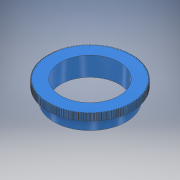
# Autodesk Inventor part: タミヤダンパー部品4
Saved by Autodesk Inventor 2020.1 (Build 241239000, 239)
## iProperties
Created: 2018-09-17
Part Number: タミヤダンパー部品4
Material: 一般
Document SubType Name: Modeling
Designer: 杉本　賢二郎
Density: 1 g/cm^3
Appearance: 既定
Author: 杉本　賢二郎
Autodesk Inventor part; units mm, degrees
(part 1 of 2)
ref_plane "YZ Plane" through (0, 0, 0) normal (1, 0, 0) x (0, 1, 0)
ref_plane "XZ Plane" through (0, 0, 0) normal (0, 1, 0) x (-1, 0, 0)
ref_plane "XY Plane" through (0, 0, 0) normal (0, 0, 1) x (1, 0, 0)
sketch "スケッチ1" plane through (0, 0, 0) normal (0, 1, 0) x (-1, 0, 0)
  line L0 (6.6972, 6.0123) -> (6.6034, 5.8356)
  arc A0 (6.8569, 5.8295) -> (6.6972, 6.0123) centre (0, 0) ccw
  line L1 (6.6692, 5.7603) -> (6.8569, 5.8295)
  arc A1 (6.6692, 5.7603) -> (6.6034, 5.8356) centre (0, 0) ccw
  line L2 (6.4207, 6.3067) -> (6.335, 6.126)
  arc A2 (6.5885, 6.1313) -> (6.4207, 6.3067) centre (0, 0) ccw
  line L3 (6.4041, 6.0538) -> (6.5885, 6.1313)
  arc A3 (6.4041, 6.0538) -> (6.335, 6.126) centre (0, 0) ccw
  line L4 (6.1313, 6.5885) -> (6.0538, 6.4041)
  arc A4 (6.3067, 6.4207) -> (6.1313, 6.5885) centre (0, 0) ccw
  line L5 (6.126, 6.335) -> (6.3067, 6.4207)
  arc A5 (6.126, 6.335) -> (6.0538, 6.4041) centre (0, 0) ccw
  line L6 (5.8295, 6.8569) -> (5.7603, 6.6692)
  arc A6 (6.0123, 6.6972) -> (5.8295, 6.8569) centre (0, 0) ccw
  line L7 (5.8356, 6.6034) -> (6.0123, 6.6972)
  arc A7 (5.8356, 6.6034) -> (5.7603, 6.6692) centre (0, 0) ccw
  line L8 (5.516, 7.1115) -> (5.4553, 6.921)
  arc A8 (5.7058, 6.9602) -> (5.516, 7.1115) centre (0, 0) ccw
  line L9 (5.5335, 6.8586) -> (5.7058, 6.9602)
  arc A9 (5.5335, 6.8586) -> (5.4553, 6.921) centre (0, 0) ccw
  line L10 (5.1914, 7.3518) -> (5.1393, 7.1587)
  arc A10 (5.3878, 7.2091) -> (5.1914, 7.3518) centre (0, 0) ccw
  line L11 (5.2202, 7.1) -> (5.3878, 7.2091)
  arc A11 (5.2202, 7.1) -> (5.1393, 7.1587) centre (0, 0) ccw
  line L12 (4.8563, 7.5774) -> (4.813, 7.3821)
  arc A12 (5.0589, 7.4436) -> (4.8563, 7.5774) centre (0, 0) ccw
  line L13 (4.8964, 7.327) -> (5.0589, 7.4436)
  arc A13 (4.8964, 7.327) -> (4.813, 7.3821) centre (0, 0) ccw
  line L14 (4.5115, 7.7876) -> (4.4769, 7.5906)
  arc A14 (4.7199, 7.6631) -> (4.5115, 7.7876) centre (0, 0) ccw
  line L15 (4.5628, 7.5393) -> (4.7199, 7.6631)
  arc A15 (4.5628, 7.5393) -> (4.4769, 7.5906) centre (0, 0) ccw
  line L16 (4.1575, 7.9822) -> (4.1319, 7.7838)
  arc A16 (4.3713, 7.8671) -> (4.1575, 7.9822) centre (0, 0) ccw
  line L17 (4.2199, 7.7364) -> (4.3713, 7.8671)
  arc A17 (4.2199, 7.7364) -> (4.1319, 7.7838) centre (0, 0) ccw
  line L18 (3.7952, 8.1607) -> (3.7785, 7.9614)
  arc A18 (4.014, 8.0553) -> (3.7952, 8.1607) centre (0, 0) ccw
  line L19 (3.8686, 7.918) -> (4.014, 8.0553)
  arc A19 (3.8686, 7.918) -> (3.7785, 7.9614) centre (0, 0) ccw
  line L20 (3.4253, 8.3227) -> (3.4175, 8.1229)
  arc A20 (3.6485, 8.2273) -> (3.4253, 8.3227) centre (0, 0) ccw
  line L21 (3.5095, 8.0836) -> (3.6485, 8.2273)
  arc A21 (3.5095, 8.0836) -> (3.4175, 8.1229) centre (0, 0) ccw
  line L22 (3.0484, 8.468) -> (3.0496, 8.268)
  arc A22 (3.2757, 8.3827) -> (3.0484, 8.468) centre (0, 0) ccw
  line L23 (3.1433, 8.2329) -> (3.2757, 8.3827)
  arc A23 (3.1433, 8.2329) -> (3.0496, 8.268) centre (0, 0) ccw
  line L24 (2.6654, 8.5962) -> (2.6756, 8.3965)
  arc A24 (2.8964, 8.5212) -> (2.6654, 8.5962) centre (0, 0) ccw
  line L25 (2.7707, 8.3656) -> (2.8964, 8.5212)
  arc A25 (2.7707, 8.3656) -> (2.6756, 8.3965) centre (0, 0) ccw
  line L26 (2.2771, 8.7072) -> (2.2962, 8.5081)
  arc A26 (2.5111, 8.6426) -> (2.2771, 8.7072) centre (0, 0) ccw
  line L27 (2.3926, 8.4815) -> (2.5111, 8.6426)
  arc A27 (2.3926, 8.4815) -> (2.2962, 8.5081) centre (0, 0) ccw
  line L28 (1.8842, 8.8006) -> (1.9122, 8.6025)
  arc A28 (2.1209, 8.7465) -> (1.8842, 8.8006) centre (0, 0) ccw
  line L29 (2.0097, 8.5803) -> (2.1209, 8.7465)
  arc A29 (2.0097, 8.5803) -> (1.9122, 8.6025) centre (0, 0) ccw
  line L30 (1.4874, 8.8762) -> (1.5243, 8.6797)
  arc A30 (1.7263, 8.8329) -> (1.4874, 8.8762) centre (0, 0) ccw
  line L31 (1.6227, 8.6618) -> (1.7263, 8.8329)
  arc A31 (1.6227, 8.6618) -> (1.5243, 8.6797) centre (0, 0) ccw
  line L32 (1.0877, 8.934) -> (1.1334, 8.7393)
  arc A32 (1.3283, 8.9014) -> (1.0877, 8.934) centre (0, 0) ccw
  line L33 (1.2325, 8.7259) -> (1.3283, 8.9014)
  arc A33 (1.2325, 8.7259) -> (1.1334, 8.7393) centre (0, 0) ccw
  line L34 (0.6858, 8.9738) -> (0.7401, 8.7814)
  arc A34 (0.9276, 8.9521) -> (0.6858, 8.9738) centre (0, 0) ccw
  line L35 (0.8397, 8.7724) -> (0.9276, 8.9521)
  arc A35 (0.8397, 8.7724) -> (0.7401, 8.7814) centre (0, 0) ccw
  line L36 (0.2825, 8.9956) -> (0.3454, 8.8057)
  arc A36 (0.525, 8.9847) -> (0.2825, 8.9956) centre (0, 0) ccw
  line L37 (0.4453, 8.8012) -> (0.525, 8.9847)
  arc A37 (0.4453, 8.8012) -> (0.3454, 8.8057) centre (0, 0) ccw
  line L38 (-0.1214, 8.9992) -> (-0.05, 8.8124)
  arc A38 (0.1214, 8.9992) -> (-0.1214, 8.9992) centre (0, 0) ccw
  line L39 (0.05, 8.8124) -> (0.1214, 8.9992)
  arc A39 (0.05, 8.8124) -> (-0.05, 8.8124) centre (0, 0) ccw
  line L40 (-0.525, 8.9847) -> (-0.4453, 8.8012)
  arc A40 (-0.2825, 8.9956) -> (-0.525, 8.9847) centre (0, 0) ccw
  line L41 (-0.3454, 8.8057) -> (-0.2825, 8.9956)
  arc A41 (-0.3454, 8.8057) -> (-0.4453, 8.8012) centre (0, 0) ccw
  line L42 (-0.9276, 8.9521) -> (-0.8397, 8.7724)
  arc A42 (-0.6858, 8.9738) -> (-0.9276, 8.9521) centre (0, 0) ccw
  line L43 (-0.7401, 8.7814) -> (-0.6858, 8.9738)
  arc A43 (-0.7401, 8.7814) -> (-0.8397, 8.7724) centre (0, 0) ccw
  line L44 (-1.3283, 8.9014) -> (-1.2325, 8.7259)
  arc A44 (-1.0877, 8.934) -> (-1.3283, 8.9014) centre (0, 0) ccw
  line L45 (-1.1334, 8.7393) -> (-1.0877, 8.934)
  arc A45 (-1.1334, 8.7393) -> (-1.2325, 8.7259) centre (0, 0) ccw
  line L46 (-1.7263, 8.8329) -> (-1.6227, 8.6618)
  arc A46 (-1.4874, 8.8762) -> (-1.7263, 8.8329) centre (0, 0) ccw
  line L47 (-1.5243, 8.6797) -> (-1.4874, 8.8762)
  arc A47 (-1.5243, 8.6797) -> (-1.6227, 8.6618) centre (0, 0) ccw
  line L48 (-2.1209, 8.7465) -> (-2.0097, 8.5803)
  arc A48 (-1.8842, 8.8006) -> (-2.1209, 8.7465) centre (0, 0) ccw
  line L49 (-1.9122, 8.6025) -> (-1.8842, 8.8006)
  arc A49 (-1.9122, 8.6025) -> (-2.0097, 8.5803) centre (0, 0) ccw
  line L50 (-2.5111, 8.6426) -> (-2.3926, 8.4815)
  arc A50 (-2.2771, 8.7072) -> (-2.5111, 8.6426) centre (0, 0) ccw
  line L51 (-2.2962, 8.5081) -> (-2.2771, 8.7072)
  arc A51 (-2.2962, 8.5081) -> (-2.3926, 8.4815) centre (0, 0) ccw
  line L52 (-2.8964, 8.5212) -> (-2.7707, 8.3656)
  arc A52 (-2.6654, 8.5962) -> (-2.8964, 8.5212) centre (0, 0) ccw
  line L53 (-2.6756, 8.3965) -> (-2.6654, 8.5962)
  arc A53 (-2.6756, 8.3965) -> (-2.7707, 8.3656) centre (0, 0) ccw
  line L54 (-3.2757, 8.3827) -> (-3.1433, 8.2329)
  arc A54 (-3.0484, 8.468) -> (-3.2757, 8.3827) centre (0, 0) ccw
  line L55 (-3.0496, 8.268) -> (-3.0484, 8.468)
  arc A55 (-3.0496, 8.268) -> (-3.1433, 8.2329) centre (0, 0) ccw
  line L56 (-3.6485, 8.2273) -> (-3.5095, 8.0836)
  arc A56 (-3.4253, 8.3227) -> (-3.6485, 8.2273) centre (0, 0) ccw
  line L57 (-3.4175, 8.1229) -> (-3.4253, 8.3227)
  arc A57 (-3.4175, 8.1229) -> (-3.5095, 8.0836) centre (0, 0) ccw
  line L58 (-4.014, 8.0553) -> (-3.8686, 7.918)
  arc A58 (-3.7952, 8.1607) -> (-4.014, 8.0553) centre (0, 0) ccw
  line L59 (-3.7785, 7.9614) -> (-3.7952, 8.1607)
  arc A59 (-3.7785, 7.9614) -> (-3.8686, 7.918) centre (0, 0) ccw
  line L60 (-4.3713, 7.8671) -> (-4.2199, 7.7364)
  arc A60 (-4.1575, 7.9822) -> (-4.3713, 7.8671) centre (0, 0) ccw
  line L61 (-4.1319, 7.7838) -> (-4.1575, 7.9822)
  arc A61 (-4.1319, 7.7838) -> (-4.2199, 7.7364) centre (0, 0) ccw
  line L62 (-4.7199, 7.6631) -> (-4.5628, 7.5393)
  arc A62 (-4.5115, 7.7876) -> (-4.7199, 7.6631) centre (0, 0) ccw
  line L63 (-4.4769, 7.5906) -> (-4.5115, 7.7876)
  arc A63 (-4.4769, 7.5906) -> (-4.5628, 7.5393) centre (0, 0) ccw
  line L64 (-5.0589, 7.4436) -> (-4.8964, 7.327)
  arc A64 (-4.8563, 7.5774) -> (-5.0589, 7.4436) centre (0, 0) ccw
  line L65 (-4.813, 7.3821) -> (-4.8563, 7.5774)
  arc A65 (-4.813, 7.3821) -> (-4.8964, 7.327) centre (0, 0) ccw
  line L66 (-5.3878, 7.2091) -> (-5.2202, 7.1)
  arc A66 (-5.1914, 7.3518) -> (-5.3878, 7.2091) centre (0, 0) ccw
  line L67 (-5.1393, 7.1587) -> (-5.1914, 7.3518)
  arc A67 (-5.1393, 7.1587) -> (-5.2202, 7.1) centre (0, 0) ccw
  line L68 (-5.7058, 6.9602) -> (-5.5335, 6.8586)
  arc A68 (-5.516, 7.1115) -> (-5.7058, 6.9602) centre (0, 0) ccw
  line L69 (-5.4553, 6.921) -> (-5.516, 7.1115)
  arc A69 (-5.4553, 6.921) -> (-5.5335, 6.8586) centre (0, 0) ccw
  line L70 (-6.0123, 6.6972) -> (-5.8356, 6.6034)
  arc A70 (-5.8295, 6.8569) -> (-6.0123, 6.6972) centre (0, 0) ccw
  line L71 (-5.7603, 6.6692) -> (-5.8295, 6.8569)
  arc A71 (-5.7603, 6.6692) -> (-5.8356, 6.6034) centre (0, 0) ccw
  line L72 (-6.3067, 6.4207) -> (-6.126, 6.335)
  arc A72 (-6.1313, 6.5885) -> (-6.3067, 6.4207) centre (0, 0) ccw
  line L73 (-6.0538, 6.4041) -> (-6.1313, 6.5885)
  arc A73 (-6.0538, 6.4041) -> (-6.126, 6.335) centre (0, 0) ccw
  line L74 (-6.5885, 6.1313) -> (-6.4041, 6.0538)
  arc A74 (-6.4207, 6.3067) -> (-6.5885, 6.1313) centre (0, 0) ccw
  line L75 (-6.335, 6.126) -> (-6.4207, 6.3067)
  arc A75 (-6.335, 6.126) -> (-6.4041, 6.0538) centre (0, 0) ccw
  line L76 (-6.8569, 5.8295) -> (-6.6692, 5.7603)
  arc A76 (-6.6972, 6.0123) -> (-6.8569, 5.8295) centre (0, 0) ccw
  line L77 (-6.6034, 5.8356) -> (-6.6972, 6.0123)
  arc A77 (-6.6034, 5.8356) -> (-6.6692, 5.7603) centre (0, 0) ccw
  line L78 (7.5774, -4.8563) -> (7.3821, -4.813)
  arc A78 (7.4436, -5.0589) -> (7.5774, -4.8563) centre (0, 0) ccw
  line L79 (7.327, -4.8964) -> (7.4436, -5.0589)
  arc A79 (7.327, -4.8964) -> (7.3821, -4.813) centre (0, 0) ccw
  line L80 (7.7876, -4.5115) -> (7.5906, -4.4769)
  arc A80 (7.6631, -4.7199) -> (7.7876, -4.5115) centre (0, 0) ccw
  line L81 (7.5393, -4.5628) -> (7.6631, -4.7199)
  arc A81 (7.5393, -4.5628) -> (7.5906, -4.4769) centre (0, 0) ccw
  line L82 (7.9822, -4.1575) -> (7.7838, -4.1319)
  arc A82 (7.8671, -4.3713) -> (7.9822, -4.1575) centre (0, 0) ccw
  line L83 (7.7364, -4.2199) -> (7.8671, -4.3713)
  arc A83 (7.7364, -4.2199) -> (7.7838, -4.1319) centre (0, 0) ccw
  line L84 (8.1607, -3.7952) -> (7.9614, -3.7785)
  arc A84 (8.0553, -4.014) -> (8.1607, -3.7952) centre (0, 0) ccw
  line L85 (7.918, -3.8686) -> (8.0553, -4.014)
  arc A85 (7.918, -3.8686) -> (7.9614, -3.7785) centre (0, 0) ccw
  line L86 (8.3227, -3.4253) -> (8.1229, -3.4175)
  arc A86 (8.2273, -3.6485) -> (8.3227, -3.4253) centre (0, 0) ccw
  line L87 (8.0836, -3.5095) -> (8.2273, -3.6485)
  arc A87 (8.0836, -3.5095) -> (8.1229, -3.4175) centre (0, 0) ccw
  line L88 (8.468, -3.0484) -> (8.268, -3.0496)
  arc A88 (8.3827, -3.2757) -> (8.468, -3.0484) centre (0, 0) ccw
  line L89 (8.2329, -3.1433) -> (8.3827, -3.2757)
  arc A89 (8.2329, -3.1433) -> (8.268, -3.0496) centre (0, 0) ccw
  line L90 (8.5962, -2.6654) -> (8.3965, -2.6756)
  arc A90 (8.5212, -2.8964) -> (8.5962, -2.6654) centre (0, 0) ccw
  line L91 (8.3656, -2.7707) -> (8.5212, -2.8964)
  arc A91 (8.3656, -2.7707) -> (8.3965, -2.6756) centre (0, 0) ccw
  line L92 (8.7072, -2.2771) -> (8.5081, -2.2962)
  arc A92 (8.6426, -2.5111) -> (8.7072, -2.2771) centre (0, 0) ccw
  line L93 (8.4815, -2.3926) -> (8.6426, -2.5111)
  arc A93 (8.4815, -2.3926) -> (8.5081, -2.2962) centre (0, 0) ccw
  line L94 (8.8006, -1.8842) -> (8.6025, -1.9122)
  arc A94 (8.7465, -2.1209) -> (8.8006, -1.8842) centre (0, 0) ccw
  line L95 (8.5803, -2.0097) -> (8.7465, -2.1209)
  arc A95 (8.5803, -2.0097) -> (8.6025, -1.9122) centre (0, 0) ccw
  line L96 (8.8762, -1.4874) -> (8.6797, -1.5243)
  arc A96 (8.8329, -1.7263) -> (8.8762, -1.4874) centre (0, 0) ccw
  line L97 (8.6618, -1.6227) -> (8.8329, -1.7263)
  arc A97 (8.6618, -1.6227) -> (8.6797, -1.5243) centre (0, 0) ccw
  line L98 (8.934, -1.0877) -> (8.7393, -1.1334)
  arc A98 (8.9014, -1.3283) -> (8.934, -1.0877) centre (0, 0) ccw
  line L99 (8.7259, -1.2325) -> (8.9014, -1.3283)
  arc A99 (8.7259, -1.2325) -> (8.7393, -1.1334) centre (0, 0) ccw
  line L100 (8.9738, -0.6858) -> (8.7814, -0.7401)
  arc A100 (8.9521, -0.9276) -> (8.9738, -0.6858) centre (0, 0) ccw
  line L101 (8.7724, -0.8397) -> (8.9521, -0.9276)
  arc A101 (8.7724, -0.8397) -> (8.7814, -0.7401) centre (0, 0) ccw
  line L102 (8.9956, -0.2825) -> (8.8057, -0.3454)
  arc A102 (8.9847, -0.525) -> (8.9956, -0.2825) centre (0, 0) ccw
  line L103 (8.8012, -0.4453) -> (8.9847, -0.525)
  arc A103 (8.8012, -0.4453) -> (8.8057, -0.3454) centre (0, 0) ccw
  line L104 (8.9992, 0.1214) -> (8.8124, 0.05)
  arc A104 (8.9992, -0.1214) -> (8.9992, 0.1214) centre (0, 0) ccw
  line L105 (8.8124, -0.05) -> (8.9992, -0.1214)
  arc A105 (8.8124, -0.05) -> (8.8124, 0.05) centre (0, 0) ccw
  line L106 (8.9847, 0.525) -> (8.8012, 0.4453)
  arc A106 (8.9956, 0.2825) -> (8.9847, 0.525) centre (0, 0) ccw
  line L107 (8.8057, 0.3454) -> (8.9956, 0.2825)
  arc A107 (8.8057, 0.3454) -> (8.8012, 0.4453) centre (0, 0) ccw
  line L108 (8.9521, 0.9276) -> (8.7724, 0.8397)
  arc A108 (8.9738, 0.6858) -> (8.9521, 0.9276) centre (0, 0) ccw
  line L109 (8.7814, 0.7401) -> (8.9738, 0.6858)
  arc A109 (8.7814, 0.7401) -> (8.7724, 0.8397) centre (0, 0) ccw
  line L110 (8.9014, 1.3283) -> (8.7259, 1.2325)
  arc A110 (8.934, 1.0877) -> (8.9014, 1.3283) centre (0, 0) ccw
  line L111 (8.7393, 1.1334) -> (8.934, 1.0877)
  arc A111 (8.7393, 1.1334) -> (8.7259, 1.2325) centre (0, 0) ccw
  line L112 (8.8329, 1.7263) -> (8.6618, 1.6227)
  arc A112 (8.8762, 1.4874) -> (8.8329, 1.7263) centre (0, 0) ccw
  line L113 (8.6797, 1.5243) -> (8.8762, 1.4874)
  arc A113 (8.6797, 1.5243) -> (8.6618, 1.6227) centre (0, 0) ccw
  line L114 (8.7465, 2.1209) -> (8.5803, 2.0097)
  arc A114 (8.8006, 1.8842) -> (8.7465, 2.1209) centre (0, 0) ccw
  line L115 (8.6025, 1.9122) -> (8.8006, 1.8842)
  arc A115 (8.6025, 1.9122) -> (8.5803, 2.0097) centre (0, 0) ccw
  line L116 (8.6426, 2.5111) -> (8.4815, 2.3926)
  arc A116 (8.7072, 2.2771) -> (8.6426, 2.5111) centre (0, 0) ccw
  line L117 (8.5081, 2.2962) -> (8.7072, 2.2771)
  arc A117 (8.5081, 2.2962) -> (8.4815, 2.3926) centre (0, 0) ccw
  line L118 (8.5212, 2.8964) -> (8.3656, 2.7707)
  arc A118 (8.5962, 2.6654) -> (8.5212, 2.8964) centre (0, 0) ccw
  line L119 (8.3965, 2.6756) -> (8.5962, 2.6654)
  arc A119 (8.3965, 2.6756) -> (8.3656, 2.7707) centre (0, 0) ccw
  line L120 (8.3827, 3.2757) -> (8.2329, 3.1433)
  arc A120 (8.468, 3.0484) -> (8.3827, 3.2757) centre (0, 0) ccw
  line L121 (8.268, 3.0496) -> (8.468, 3.0484)
  arc A121 (8.268, 3.0496) -> (8.2329, 3.1433) centre (0, 0) ccw
  line L122 (8.2273, 3.6485) -> (8.0836, 3.5095)
  arc A122 (8.3227, 3.4253) -> (8.2273, 3.6485) centre (0, 0) ccw
  line L123 (8.1229, 3.4175) -> (8.3227, 3.4253)
  arc A123 (8.1229, 3.4175) -> (8.0836, 3.5095) centre (0, 0) ccw
  line L124 (8.0553, 4.014) -> (7.918, 3.8686)
  arc A124 (8.1607, 3.7952) -> (8.0553, 4.014) centre (0, 0) ccw
  line L125 (7.9614, 3.7785) -> (8.1607, 3.7952)
  arc A125 (7.9614, 3.7785) -> (7.918, 3.8686) centre (0, 0) ccw
  line L126 (7.8671, 4.3713) -> (7.7364, 4.2199)
  arc A126 (7.9822, 4.1575) -> (7.8671, 4.3713) centre (0, 0) ccw
  line L127 (7.7838, 4.1319) -> (7.9822, 4.1575)
  arc A127 (7.7838, 4.1319) -> (7.7364, 4.2199) centre (0, 0) ccw
  line L128 (7.6631, 4.7199) -> (7.5393, 4.5628)
  arc A128 (7.7876, 4.5115) -> (7.6631, 4.7199) centre (0, 0) ccw
  line L129 (7.5906, 4.4769) -> (7.7876, 4.5115)
  arc A129 (7.5906, 4.4769) -> (7.5393, 4.5628) centre (0, 0) ccw
  line L130 (7.4436, 5.0589) -> (7.327, 4.8964)
  arc A130 (7.5774, 4.8563) -> (7.4436, 5.0589) centre (0, 0) ccw
  line L131 (7.3821, 4.813) -> (7.5774, 4.8563)
  arc A131 (7.3821, 4.813) -> (7.327, 4.8964) centre (0, 0) ccw
  line L132 (7.2091, 5.3878) -> (7.1, 5.2202)
  arc A132 (7.3518, 5.1914) -> (7.2091, 5.3878) centre (0, 0) ccw
  line L133 (7.1587, 5.1393) -> (7.3518, 5.1914)
  arc A133 (7.1587, 5.1393) -> (7.1, 5.2202) centre (0, 0) ccw
  line L134 (6.9602, 5.7058) -> (6.8586, 5.5335)
  arc A134 (7.1115, 5.516) -> (6.9602, 5.7058) centre (0, 0) ccw
  line L135 (6.921, 5.4553) -> (7.1115, 5.516)
  arc A135 (6.921, 5.4553) -> (6.8586, 5.5335) centre (0, 0) ccw
  line L136 (6.6972, 6.0123) -> (6.6034, 5.8356)
  arc A136 (6.8569, 5.8295) -> (6.6972, 6.0123) centre (0, 0) ccw
  line L137 (6.6692, 5.7603) -> (6.8569, 5.8295)
  arc A137 (6.6692, 5.7603) -> (6.6034, 5.8356) centre (0, 0) ccw
  line L138 (6.4207, 6.3067) -> (6.335, 6.126)
  arc A138 (6.5885, 6.1313) -> (6.4207, 6.3067) centre (0, 0) ccw
  line L139 (6.4041, 6.0538) -> (6.5885, 6.1313)
  arc A139 (6.4041, 6.0538) -> (6.335, 6.126) centre (0, 0) ccw
  line L140 (6.1313, 6.5885) -> (6.0538, 6.4041)
  arc A140 (6.3067, 6.4207) -> (6.1313, 6.5885) centre (0, 0) ccw
  line L141 (6.126, 6.335) -> (6.3067, 6.4207)
  arc A141 (6.126, 6.335) -> (6.0538, 6.4041) centre (0, 0) ccw
  line L142 (5.8295, 6.8569) -> (5.7603, 6.6692)
  arc A142 (6.0123, 6.6972) -> (5.8295, 6.8569) centre (0, 0) ccw
  line L143 (5.8356, 6.6034) -> (6.0123, 6.6972)
  arc A143 (5.8356, 6.6034) -> (5.7603, 6.6692) centre (0, 0) ccw
  line L144 (5.516, 7.1115) -> (5.4553, 6.921)
  arc A144 (5.7058, 6.9602) -> (5.516, 7.1115) centre (0, 0) ccw
  line L145 (5.5335, 6.8586) -> (5.7058, 6.9602)
  arc A145 (5.5335, 6.8586) -> (5.4553, 6.921) centre (0, 0) ccw
  line L146 (5.1914, 7.3518) -> (5.1393, 7.1587)
  arc A146 (5.3878, 7.2091) -> (5.1914, 7.3518) centre (0, 0) ccw
  line L147 (5.2202, 7.1) -> (5.3878, 7.2091)
  arc A147 (5.2202, 7.1) -> (5.1393, 7.1587) centre (0, 0) ccw
  line L148 (4.8563, 7.5774) -> (4.813, 7.3821)
  arc A148 (5.0589, 7.4436) -> (4.8563, 7.5774) centre (0, 0) ccw
  line L149 (4.8964, 7.327) -> (5.0589, 7.4436)
  arc A149 (4.8964, 7.327) -> (4.813, 7.3821) centre (0, 0) ccw
  line L150 (4.5115, 7.7876) -> (4.4769, 7.5906)
  arc A150 (4.7199, 7.6631) -> (4.5115, 7.7876) centre (0, 0) ccw
  line L151 (4.5628, 7.5393) -> (4.7199, 7.6631)
  arc A151 (4.5628, 7.5393) -> (4.4769, 7.5906) centre (0, 0) ccw
  line L152 (4.1575, 7.9822) -> (4.1319, 7.7838)
  arc A152 (4.3713, 7.8671) -> (4.1575, 7.9822) centre (0, 0) ccw
  line L153 (4.2199, 7.7364) -> (4.3713, 7.8671)
  arc A153 (4.2199, 7.7364) -> (4.1319, 7.7838) centre (0, 0) ccw
  line L154 (3.7952, 8.1607) -> (3.7785, 7.9614)
  line L155 (3.8686, 7.918) -> (4.014, 8.0553)
  arc A154 (3.8686, 7.918) -> (3.7785, 7.9614) centre (0, 0) ccw
  line L156 (1.7263, -8.8329) -> (1.6227, -8.6618)
  arc A155 (1.4874, -8.8762) -> (1.7263, -8.8329) centre (0, 0) ccw
  line L157 (1.5243, -8.6797) -> (1.4874, -8.8762)
  arc A156 (1.5243, -8.6797) -> (1.6227, -8.6618) centre (0, 0) ccw
  line L158 (2.1209, -8.7465) -> (2.0097, -8.5803)
  arc A157 (1.8842, -8.8006) -> (2.1209, -8.7465) centre (0, 0) ccw
  line L159 (1.9122, -8.6025) -> (1.8842, -8.8006)
  arc A158 (1.9122, -8.6025) -> (2.0097, -8.5803) centre (0, 0) ccw
  line L160 (2.5111, -8.6426) -> (2.3926, -8.4815)
  arc A159 (2.2771, -8.7072) -> (2.5111, -8.6426) centre (0, 0) ccw
  line L161 (2.2962, -8.5081) -> (2.2771, -8.7072)
  arc A160 (2.2962, -8.5081) -> (2.3926, -8.4815) centre (0, 0) ccw
  line L162 (2.8964, -8.5212) -> (2.7707, -8.3656)
  arc A161 (2.6654, -8.5962) -> (2.8964, -8.5212) centre (0, 0) ccw
  line L163 (2.6756, -8.3965) -> (2.6654, -8.5962)
  arc A162 (2.6756, -8.3965) -> (2.7707, -8.3656) centre (0, 0) ccw
  line L164 (3.2757, -8.3827) -> (3.1433, -8.2329)
  arc A163 (3.0484, -8.468) -> (3.2757, -8.3827) centre (0, 0) ccw
  line L165 (3.0496, -8.268) -> (3.0484, -8.468)
  arc A164 (3.0496, -8.268) -> (3.1433, -8.2329) centre (0, 0) ccw
  line L166 (3.6485, -8.2273) -> (3.5095, -8.0836)
  arc A165 (3.4253, -8.3227) -> (3.6485, -8.2273) centre (0, 0) ccw
  line L167 (3.4175, -8.1229) -> (3.4253, -8.3227)
  arc A166 (3.4175, -8.1229) -> (3.5095, -8.0836) centre (0, 0) ccw
  line L168 (4.014, -8.0553) -> (3.8686, -7.918)
  arc A167 (3.7952, -8.1607) -> (4.014, -8.0553) centre (0, 0) ccw
  line L169 (3.7785, -7.9614) -> (3.7952, -8.1607)
  arc A168 (3.7785, -7.9614) -> (3.8686, -7.918) centre (0, 0) ccw
  line L170 (4.3713, -7.8671) -> (4.2199, -7.7364)
  arc A169 (4.1575, -7.9822) -> (4.3713, -7.8671) centre (0, 0) ccw
  line L171 (4.1319, -7.7838) -> (4.1575, -7.9822)
  arc A170 (4.1319, -7.7838) -> (4.2199, -7.7364) centre (0, 0) ccw
  line L172 (4.7199, -7.6631) -> (4.5628, -7.5393)
  arc A171 (4.5115, -7.7876) -> (4.7199, -7.6631) centre (0, 0) ccw
  line L173 (4.4769, -7.5906) -> (4.5115, -7.7876)
  arc A172 (4.4769, -7.5906) -> (4.5628, -7.5393) centre (0, 0) ccw
  line L174 (5.0589, -7.4436) -> (4.8964, -7.327)
  arc A173 (4.8563, -7.5774) -> (5.0589, -7.4436) centre (0, 0) ccw
  line L175 (4.813, -7.3821) -> (4.8563, -7.5774)
  arc A174 (4.813, -7.3821) -> (4.8964, -7.327) centre (0, 0) ccw
  line L176 (5.3878, -7.2091) -> (5.2202, -7.1)
  arc A175 (5.1914, -7.3518) -> (5.3878, -7.2091) centre (0, 0) ccw
  line L177 (5.1393, -7.1587) -> (5.1914, -7.3518)
  arc A176 (5.1393, -7.1587) -> (5.2202, -7.1) centre (0, 0) ccw
  line L178 (5.7058, -6.9602) -> (5.5335, -6.8586)
  arc A177 (5.516, -7.1115) -> (5.7058, -6.9602) centre (0, 0) ccw
  line L179 (5.4553, -6.921) -> (5.516, -7.1115)
  arc A178 (5.4553, -6.921) -> (5.5335, -6.8586) centre (0, 0) ccw
  line L180 (6.0123, -6.6972) -> (5.8356, -6.6034)
  arc A179 (5.8295, -6.8569) -> (6.0123, -6.6972) centre (0, 0) ccw
  line L181 (5.7603, -6.6692) -> (5.8295, -6.8569)
  arc A180 (5.7603, -6.6692) -> (5.8356, -6.6034) centre (0, 0) ccw
  line L182 (6.3067, -6.4207) -> (6.126, -6.335)
  arc A181 (6.1313, -6.5885) -> (6.3067, -6.4207) centre (0, 0) ccw
  line L183 (6.0538, -6.4041) -> (6.1313, -6.5885)
  arc A182 (6.0538, -6.4041) -> (6.126, -6.335) centre (0, 0) ccw
  line L184 (6.5885, -6.1313) -> (6.4041, -6.0538)
  arc A183 (6.4207, -6.3067) -> (6.5885, -6.1313) centre (0, 0) ccw
  line L185 (6.335, -6.126) -> (6.4207, -6.3067)
  arc A184 (6.335, -6.126) -> (6.4041, -6.0538) centre (0, 0) ccw
  line L186 (6.8569, -5.8295) -> (6.6692, -5.7603)
  arc A185 (6.6972, -6.0123) -> (6.8569, -5.8295) centre (0, 0) ccw
  line L187 (6.6034, -5.8356) -> (6.6972, -6.0123)
  arc A186 (6.6034, -5.8356) -> (6.6692, -5.7603) centre (0, 0) ccw
  line L188 (7.1115, -5.516) -> (6.921, -5.4553)
  arc A187 (6.9602, -5.7058) -> (7.1115, -5.516) centre (0, 0) ccw
  line L189 (6.8586, -5.5335) -> (6.9602, -5.7058)
  arc A188 (6.8586, -5.5335) -> (6.921, -5.4553) centre (0, 0) ccw
  line L190 (7.3518, -5.1914) -> (7.1587, -5.1393)
  arc A189 (7.2091, -5.3878) -> (7.3518, -5.1914) centre (0, 0) ccw
  line L191 (7.1, -5.2202) -> (7.2091, -5.3878)
  arc A190 (7.1, -5.2202) -> (7.1587, -5.1393) centre (0, 0) ccw
  line L192 (7.5774, -4.8563) -> (7.3821, -4.813)
  arc A191 (7.4436, -5.0589) -> (7.5774, -4.8563) centre (0, 0) ccw
  line L193 (7.327, -4.8964) -> (7.4436, -5.0589)
  arc A192 (7.327, -4.8964) -> (7.3821, -4.813) centre (0, 0) ccw
  line L194 (7.7876, -4.5115) -> (7.5906, -4.4769)
  arc A193 (7.6631, -4.7199) -> (7.7876, -4.5115) centre (0, 0) ccw
  line L195 (7.5393, -4.5628) -> (7.6631, -4.7199)
  arc A194 (7.5393, -4.5628) -> (7.5906, -4.4769) centre (0, 0) ccw
  line L196 (7.9822, -4.1575) -> (7.7838, -4.1319)
  arc A195 (7.8671, -4.3713) -> (7.9822, -4.1575) centre (0, 0) ccw
  line L197 (7.7364, -4.2199) -> (7.8671, -4.3713)
  arc A196 (7.7364, -4.2199) -> (7.7838, -4.1319) centre (0, 0) ccw
  line L198 (8.1607, -3.7952) -> (7.9614, -3.7785)
  arc A197 (8.0553, -4.014) -> (8.1607, -3.7952) centre (0, 0) ccw
  line L199 (7.918, -3.8686) -> (8.0553, -4.014)
  arc A198 (7.918, -3.8686) -> (7.9614, -3.7785) centre (0, 0) ccw
  line L200 (8.3227, -3.4253) -> (8.1229, -3.4175)
  arc A199 (8.2273, -3.6485) -> (8.3227, -3.4253) centre (0, 0) ccw
  line L201 (8.0836, -3.5095) -> (8.2273, -3.6485)
  arc A200 (8.0836, -3.5095) -> (8.1229, -3.4175) centre (0, 0) ccw
  line L202 (8.468, -3.0484) -> (8.268, -3.0496)
  arc A201 (8.3827, -3.2757) -> (8.468, -3.0484) centre (0, 0) ccw
  line L203 (8.2329, -3.1433) -> (8.3827, -3.2757)
  arc A202 (8.2329, -3.1433) -> (8.268, -3.0496) centre (0, 0) ccw
  line L204 (8.5962, -2.6654) -> (8.3965, -2.6756)
  arc A203 (8.5212, -2.8964) -> (8.5962, -2.6654) centre (0, 0) ccw
  line L205 (8.3656, -2.7707) -> (8.5212, -2.8964)
  arc A204 (8.3656, -2.7707) -> (8.3965, -2.6756) centre (0, 0) ccw
  line L206 (8.7072, -2.2771) -> (8.5081, -2.2962)
  arc A205 (8.6426, -2.5111) -> (8.7072, -2.2771) centre (0, 0) ccw
  line L207 (8.4815, -2.3926) -> (8.6426, -2.5111)
  arc A206 (8.4815, -2.3926) -> (8.5081, -2.2962) centre (0, 0) ccw
  line L208 (8.8006, -1.8842) -> (8.6025, -1.9122)
  arc A207 (8.7465, -2.1209) -> (8.8006, -1.8842) centre (0, 0) ccw
  line L209 (8.5803, -2.0097) -> (8.7465, -2.1209)
  arc A208 (8.5803, -2.0097) -> (8.6025, -1.9122) centre (0, 0) ccw
  line L210 (8.8762, -1.4874) -> (8.6797, -1.5243)
  arc A209 (8.8329, -1.7263) -> (8.8762, -1.4874) centre (0, 0) ccw
  line L211 (8.6618, -1.6227) -> (8.8329, -1.7263)
  arc A210 (8.6618, -1.6227) -> (8.6797, -1.5243) centre (0, 0) ccw
  line L212 (8.934, -1.0877) -> (8.7393, -1.1334)
  arc A211 (8.9014, -1.3283) -> (8.934, -1.0877) centre (0, 0) ccw
  line L213 (8.7259, -1.2325) -> (8.9014, -1.3283)
  arc A212 (8.7259, -1.2325) -> (8.7393, -1.1334) centre (0, 0) ccw
  line L214 (8.9738, -0.6858) -> (8.7814, -0.7401)
  arc A213 (8.9521, -0.9276) -> (8.9738, -0.6858) centre (0, 0) ccw
  line L215 (8.7724, -0.8397) -> (8.9521, -0.9276)
  arc A214 (8.7724, -0.8397) -> (8.7814, -0.7401) centre (0, 0) ccw
  line L216 (8.9956, -0.2825) -> (8.8057, -0.3454)
  arc A215 (8.9847, -0.525) -> (8.9956, -0.2825) centre (0, 0) ccw
  line L217 (8.8012, -0.4453) -> (8.9847, -0.525)
  arc A216 (8.8012, -0.4453) -> (8.8057, -0.3454) centre (0, 0) ccw
  line L218 (8.9992, 0.1214) -> (8.8124, 0.05)
  arc A217 (8.9992, -0.1214) -> (8.9992, 0.1214) centre (0, 0) ccw
  line L219 (8.8124, -0.05) -> (8.9992, -0.1214)
  arc A218 (8.8124, -0.05) -> (8.8124, 0.05) centre (0, 0) ccw
  arc A219 (8.9956, 0.2825) -> (8.9847, 0.525) centre (0, 0) ccw
  line L220 (8.8057, 0.3454) -> (8.9956, 0.2825)
  arc A220 (-0.1214, -8.9992) -> (0.1214, -8.9992) centre (0, 0) ccw
  arc A221 (-0.05, -8.8124) -> (0.05, -8.8124) centre (0, 0) ccw
  line L221 (0.1214, -8.9992) -> (0.05, -8.8124)
  line L222 (-0.05, -8.8124) -> (-0.1214, -8.9992)
  line L223 (0, -8.8125) -> (0, 0)
  line L224 (0.525, -8.9847) -> (0.4453, -8.8012)
  arc A222 (0.2825, -8.9956) -> (0.525, -8.9847) centre (0, 0) ccw
  line L225 (0.3454, -8.8057) -> (0.2825, -8.9956)
  arc A223 (0.3454, -8.8057) -> (0.4453, -8.8012) centre (0, 0) ccw
  line L226 (0.9276, -8.9521) -> (0.8397, -8.7724)
  arc A224 (0.6858, -8.9738) -> (0.9276, -8.9521) centre (0, 0) ccw
  line L227 (0.7401, -8.7814) -> (0.6858, -8.9738)
  arc A225 (0.7401, -8.7814) -> (0.8397, -8.7724) centre (0, 0) ccw
  line L228 (1.3283, -8.9014) -> (1.2325, -8.7259)
  arc A226 (1.0877, -8.934) -> (1.3283, -8.9014) centre (0, 0) ccw
  line L229 (1.1334, -8.7393) -> (1.0877, -8.934)
  arc A227 (1.1334, -8.7393) -> (1.2325, -8.7259) centre (0, 0) ccw
  line L230 (1.7263, -8.8329) -> (1.6227, -8.6618)
  arc A228 (1.4874, -8.8762) -> (1.7263, -8.8329) centre (0, 0) ccw
  line L231 (1.5243, -8.6797) -> (1.4874, -8.8762)
  arc A229 (1.5243, -8.6797) -> (1.6227, -8.6618) centre (0, 0) ccw
  line L232 (2.1209, -8.7465) -> (2.0097, -8.5803)
  arc A230 (1.8842, -8.8006) -> (2.1209, -8.7465) centre (0, 0) ccw
  line L233 (1.9122, -8.6025) -> (1.8842, -8.8006)
  arc A231 (1.9122, -8.6025) -> (2.0097, -8.5803) centre (0, 0) ccw
  line L234 (2.5111, -8.6426) -> (2.3926, -8.4815)
  arc A232 (2.2771, -8.7072) -> (2.5111, -8.6426) centre (0, 0) ccw
  line L235 (2.2962, -8.5081) -> (2.2771, -8.7072)
  arc A233 (2.2962, -8.5081) -> (2.3926, -8.4815) centre (0, 0) ccw
  line L236 (-8.2273, -3.6485) -> (-8.0836, -3.5095)
  arc A234 (-8.3227, -3.4253) -> (-8.2273, -3.6485) centre (0, 0) ccw
  arc A235 (-8.1229, -3.4175) -> (-8.0836, -3.5095) centre (0, 0) ccw
  line L237 (-8.0553, -4.014) -> (-7.918, -3.8686)
  arc A236 (-8.1607, -3.7952) -> (-8.0553, -4.014) centre (0, 0) ccw
  line L238 (-7.9614, -3.7785) -> (-8.1607, -3.7952)
  arc A237 (-7.9614, -3.7785) -> (-7.918, -3.8686) centre (0, 0) ccw
  line L239 (-7.8671, -4.3713) -> (-7.7364, -4.2199)
  arc A238 (-7.9822, -4.1575) -> (-7.8671, -4.3713) centre (0, 0) ccw
  line L240 (-7.7838, -4.1319) -> (-7.9822, -4.1575)
  arc A239 (-7.7838, -4.1319) -> (-7.7364, -4.2199) centre (0, 0) ccw
  line L241 (-7.6631, -4.7199) -> (-7.5393, -4.5628)
  arc A240 (-7.7876, -4.5115) -> (-7.6631, -4.7199) centre (0, 0) ccw
  line L242 (-7.5906, -4.4769) -> (-7.7876, -4.5115)
  arc A241 (-7.5906, -4.4769) -> (-7.5393, -4.5628) centre (0, 0) ccw
  line L243 (-7.4436, -5.0589) -> (-7.327, -4.8964)
  arc A242 (-7.5774, -4.8563) -> (-7.4436, -5.0589) centre (0, 0) ccw
  line L244 (-7.3821, -4.813) -> (-7.5774, -4.8563)
  arc A243 (-7.3821, -4.813) -> (-7.327, -4.8964) centre (0, 0) ccw
  line L245 (-7.2091, -5.3878) -> (-7.1, -5.2202)
  arc A244 (-7.3518, -5.1914) -> (-7.2091, -5.3878) centre (0, 0) ccw
  line L246 (-7.1587, -5.1393) -> (-7.3518, -5.1914)
  arc A245 (-7.1587, -5.1393) -> (-7.1, -5.2202) centre (0, 0) ccw
  line L247 (-6.9602, -5.7058) -> (-6.8586, -5.5335)
  arc A246 (-7.1115, -5.516) -> (-6.9602, -5.7058) centre (0, 0) ccw
  line L248 (-6.921, -5.4553) -> (-7.1115, -5.516)
  arc A247 (-6.921, -5.4553) -> (-6.8586, -5.5335) centre (0, 0) ccw
  line L249 (-6.6972, -6.0123) -> (-6.6034, -5.8356)
  arc A248 (-6.8569, -5.8295) -> (-6.6972, -6.0123) centre (0, 0) ccw
  line L250 (-6.6692, -5.7603) -> (-6.8569, -5.8295)
  arc A249 (-6.6692, -5.7603) -> (-6.6034, -5.8356) centre (0, 0) ccw
  line L251 (-6.4207, -6.3067) -> (-6.335, -6.126)
  arc A250 (-6.5885, -6.1313) -> (-6.4207, -6.3067) centre (0, 0) ccw
  line L252 (-6.4041, -6.0538) -> (-6.5885, -6.1313)
  arc A251 (-6.4041, -6.0538) -> (-6.335, -6.126) centre (0, 0) ccw
  line L253 (-6.1313, -6.5885) -> (-6.0538, -6.4041)
  arc A252 (-6.3067, -6.4207) -> (-6.1313, -6.5885) centre (0, 0) ccw
  line L254 (-6.126, -6.335) -> (-6.3067, -6.4207)
  arc A253 (-6.126, -6.335) -> (-6.0538, -6.4041) centre (0, 0) ccw
  line L255 (-5.8295, -6.8569) -> (-5.7603, -6.6692)
  arc A254 (-6.0123, -6.6972) -> (-5.8295, -6.8569) centre (0, 0) ccw
  line L256 (-5.8356, -6.6034) -> (-6.0123, -6.6972)
  arc A255 (-5.8356, -6.6034) -> (-5.7603, -6.6692) centre (0, 0) ccw
  line L257 (-5.516, -7.1115) -> (-5.4553, -6.921)
  arc A256 (-5.7058, -6.9602) -> (-5.516, -7.1115) centre (0, 0) ccw
  line L258 (-5.5335, -6.8586) -> (-5.7058, -6.9602)
  arc A257 (-5.5335, -6.8586) -> (-5.4553, -6.921) centre (0, 0) ccw
  line L259 (-5.1914, -7.3518) -> (-5.1393, -7.1587)
  arc A258 (-5.3878, -7.2091) -> (-5.1914, -7.3518) centre (0, 0) ccw
  line L260 (-5.2202, -7.1) -> (-5.3878, -7.2091)
  arc A259 (-5.2202, -7.1) -> (-5.1393, -7.1587) centre (0, 0) ccw
  line L261 (-4.8563, -7.5774) -> (-4.813, -7.3821)
  arc A260 (-5.0589, -7.4436) -> (-4.8563, -7.5774) centre (0, 0) ccw
  line L262 (-4.8964, -7.327) -> (-5.0589, -7.4436)
  arc A261 (-4.8964, -7.327) -> (-4.813, -7.3821) centre (0, 0) ccw
  line L263 (-4.5115, -7.7876) -> (-4.4769, -7.5906)
  arc A262 (-4.7199, -7.6631) -> (-4.5115, -7.7876) centre (0, 0) ccw
  line L264 (-4.5628, -7.5393) -> (-4.7199, -7.6631)
  arc A263 (-4.5628, -7.5393) -> (-4.4769, -7.5906) centre (0, 0) ccw
  line L265 (-4.1575, -7.9822) -> (-4.1319, -7.7838)
  arc A264 (-4.3713, -7.8671) -> (-4.1575, -7.9822) centre (0, 0) ccw
  line L266 (-4.2199, -7.7364) -> (-4.3713, -7.8671)
  arc A265 (-4.2199, -7.7364) -> (-4.1319, -7.7838) centre (0, 0) ccw
  line L267 (-3.7952, -8.1607) -> (-3.7785, -7.9614)
  arc A266 (-4.014, -8.0553) -> (-3.7952, -8.1607) centre (0, 0) ccw
  line L268 (-3.8686, -7.918) -> (-4.014, -8.0553)
  arc A267 (-3.8686, -7.918) -> (-3.7785, -7.9614) centre (0, 0) ccw
  line L269 (-3.4253, -8.3227) -> (-3.4175, -8.1229)
  arc A268 (-3.6485, -8.2273) -> (-3.4253, -8.3227) centre (0, 0) ccw
  line L270 (-3.5095, -8.0836) -> (-3.6485, -8.2273)
  arc A269 (-3.5095, -8.0836) -> (-3.4175, -8.1229) centre (0, 0) ccw
  line L271 (-3.0484, -8.468) -> (-3.0496, -8.268)
  arc A270 (-3.2757, -8.3827) -> (-3.0484, -8.468) centre (0, 0) ccw
  line L272 (-3.1433, -8.2329) -> (-3.2757, -8.3827)
  arc A271 (-3.1433, -8.2329) -> (-3.0496, -8.268) centre (0, 0) ccw
  line L273 (-2.6654, -8.5962) -> (-2.6756, -8.3965)
  arc A272 (-2.8964, -8.5212) -> (-2.6654, -8.5962) centre (0, 0) ccw
  line L274 (-2.7707, -8.3656) -> (-2.8964, -8.5212)
  arc A273 (-2.7707, -8.3656) -> (-2.6756, -8.3965) centre (0, 0) ccw
  line L275 (-2.2771, -8.7072) -> (-2.2962, -8.5081)
  arc A274 (-2.5111, -8.6426) -> (-2.2771, -8.7072) centre (0, 0) ccw
  line L276 (-2.3926, -8.4815) -> (-2.5111, -8.6426)
  arc A275 (-2.3926, -8.4815) -> (-2.2962, -8.5081) centre (0, 0) ccw
  line L277 (-1.8842, -8.8006) -> (-1.9122, -8.6025)
  arc A276 (-2.1209, -8.7465) -> (-1.8842, -8.8006) centre (0, 0) ccw
  line L278 (-2.0097, -8.5803) -> (-2.1209, -8.7465)
  arc A277 (-2.0097, -8.5803) -> (-1.9122, -8.6025) centre (0, 0) ccw
  line L279 (-1.4874, -8.8762) -> (-1.5243, -8.6797)
  arc A278 (-1.7263, -8.8329) -> (-1.4874, -8.8762) centre (0, 0) ccw
  line L280 (-1.6227, -8.6618) -> (-1.7263, -8.8329)
  arc A279 (-1.6227, -8.6618) -> (-1.5243, -8.6797) centre (0, 0) ccw
  line L281 (-1.0877, -8.934) -> (-1.1334, -8.7393)
  arc A280 (-1.3283, -8.9014) -> (-1.0877, -8.934) centre (0, 0) ccw
  line L282 (-1.2325, -8.7259) -> (-1.3283, -8.9014)
  arc A281 (-1.2325, -8.7259) -> (-1.1334, -8.7393) centre (0, 0) ccw
  line L283 (-0.6858, -8.9738) -> (-0.7401, -8.7814)
  arc A282 (-0.9276, -8.9521) -> (-0.6858, -8.9738) centre (0, 0) ccw
  line L284 (-0.8397, -8.7724) -> (-0.9276, -8.9521)
  arc A283 (-0.8397, -8.7724) -> (-0.7401, -8.7814) centre (0, 0) ccw
  line L285 (-0.2825, -8.9956) -> (-0.3454, -8.8057)
  arc A284 (-0.525, -8.9847) -> (-0.2825, -8.9956) centre (0, 0) ccw
  line L286 (-0.4453, -8.8012) -> (-0.525, -8.9847)
  arc A285 (-0.4453, -8.8012) -> (-0.3454, -8.8057) centre (0, 0) ccw
  line L287 (-5.0589, 7.4436) -> (-4.8964, 7.327)
  arc A286 (-4.8563, 7.5774) -> (-5.0589, 7.4436) centre (0, 0) ccw
  line L288 (-4.813, 7.3821) -> (-4.8563, 7.5774)
  arc A287 (-4.813, 7.3821) -> (-4.8964, 7.327) centre (0, 0) ccw
  line L289 (-5.3878, 7.2091) -> (-5.2202, 7.1)
  arc A288 (-5.1914, 7.3518) -> (-5.3878, 7.2091) centre (0, 0) ccw
  line L290 (-5.1393, 7.1587) -> (-5.1914, 7.3518)
  arc A289 (-5.1393, 7.1587) -> (-5.2202, 7.1) centre (0, 0) ccw
  line L291 (-5.7058, 6.9602) -> (-5.5335, 6.8586)
  arc A290 (-5.516, 7.1115) -> (-5.7058, 6.9602) centre (0, 0) ccw
  line L292 (-5.4553, 6.921) -> (-5.516, 7.1115)
  arc A291 (-5.4553, 6.921) -> (-5.5335, 6.8586) centre (0, 0) ccw
  line L293 (-6.0123, 6.6972) -> (-5.8356, 6.6034)
  arc A292 (-5.8295, 6.8569) -> (-6.0123, 6.6972) centre (0, 0) ccw
  line L294 (-5.7603, 6.6692) -> (-5.8295, 6.8569)
  arc A293 (-5.7603, 6.6692) -> (-5.8356, 6.6034) centre (0, 0) ccw
  line L295 (-6.3067, 6.4207) -> (-6.126, 6.335)
  arc A294 (-6.1313, 6.5885) -> (-6.3067, 6.4207) centre (0, 0) ccw
  line L296 (-6.0538, 6.4041) -> (-6.1313, 6.5885)
  arc A295 (-6.0538, 6.4041) -> (-6.126, 6.335) centre (0, 0) ccw
  line L297 (-6.5885, 6.1313) -> (-6.4041, 6.0538)
  arc A296 (-6.4207, 6.3067) -> (-6.5885, 6.1313) centre (0, 0) ccw
  line L298 (-6.335, 6.126) -> (-6.4207, 6.3067)
  arc A297 (-6.335, 6.126) -> (-6.4041, 6.0538) centre (0, 0) ccw
  line L299 (-6.8569, 5.8295) -> (-6.6692, 5.7603)
  arc A298 (-6.6972, 6.0123) -> (-6.8569, 5.8295) centre (0, 0) ccw
  line L300 (-6.6034, 5.8356) -> (-6.6972, 6.0123)
  arc A299 (-6.6034, 5.8356) -> (-6.6692, 5.7603) centre (0, 0) ccw
  line L301 (-7.1115, 5.516) -> (-6.921, 5.4553)
  arc A300 (-6.9602, 5.7058) -> (-7.1115, 5.516) centre (0, 0) ccw
  line L302 (-6.8586, 5.5335) -> (-6.9602, 5.7058)
  arc A301 (-6.8586, 5.5335) -> (-6.921, 5.4553) centre (0, 0) ccw
  line L303 (-7.3518, 5.1914) -> (-7.1587, 5.1393)
  arc A302 (-7.2091, 5.3878) -> (-7.3518, 5.1914) centre (0, 0) ccw
  line L304 (-7.1, 5.2202) -> (-7.2091, 5.3878)
  arc A303 (-7.1, 5.2202) -> (-7.1587, 5.1393) centre (0, 0) ccw
  line L305 (-7.5774, 4.8563) -> (-7.3821, 4.813)
  arc A304 (-7.4436, 5.0589) -> (-7.5774, 4.8563) centre (0, 0) ccw
  line L306 (-7.327, 4.8964) -> (-7.4436, 5.0589)
  arc A305 (-7.327, 4.8964) -> (-7.3821, 4.813) centre (0, 0) ccw
  line L307 (-7.7876, 4.5115) -> (-7.5906, 4.4769)
  arc A306 (-7.6631, 4.7199) -> (-7.7876, 4.5115) centre (0, 0) ccw
  line L308 (-7.5393, 4.5628) -> (-7.6631, 4.7199)
  arc A307 (-7.5393, 4.5628) -> (-7.5906, 4.4769) centre (0, 0) ccw
  line L309 (-7.9822, 4.1575) -> (-7.7838, 4.1319)
  arc A308 (-7.8671, 4.3713) -> (-7.9822, 4.1575) centre (0, 0) ccw
  line L310 (-7.7364, 4.2199) -> (-7.8671, 4.3713)
  arc A309 (-7.7364, 4.2199) -> (-7.7838, 4.1319) centre (0, 0) ccw
  line L311 (-8.1607, 3.7952) -> (-7.9614, 3.7785)
  arc A310 (-8.0553, 4.014) -> (-8.1607, 3.7952) centre (0, 0) ccw
  line L312 (-7.918, 3.8686) -> (-8.0553, 4.014)
  arc A311 (-7.918, 3.8686) -> (-7.9614, 3.7785) centre (0, 0) ccw
  line L313 (-8.3227, 3.4253) -> (-8.1229, 3.4175)
  arc A312 (-8.2273, 3.6485) -> (-8.3227, 3.4253) centre (0, 0) ccw
  line L314 (-8.0836, 3.5095) -> (-8.2273, 3.6485)
  arc A313 (-8.0836, 3.5095) -> (-8.1229, 3.4175) centre (0, 0) ccw
  line L315 (-8.468, 3.0484) -> (-8.268, 3.0496)
  arc A314 (-8.3827, 3.2757) -> (-8.468, 3.0484) centre (0, 0) ccw
  line L316 (-8.2329, 3.1433) -> (-8.3827, 3.2757)
  arc A315 (-8.2329, 3.1433) -> (-8.268, 3.0496) centre (0, 0) ccw
  line L317 (-8.5962, 2.6654) -> (-8.3965, 2.6756)
  arc A316 (-8.5212, 2.8964) -> (-8.5962, 2.6654) centre (0, 0) ccw
  line L318 (-8.3656, 2.7707) -> (-8.5212, 2.8964)
  arc A317 (-8.3656, 2.7707) -> (-8.3965, 2.6756) centre (0, 0) ccw
  line L319 (-8.7072, 2.2771) -> (-8.5081, 2.2962)
  arc A318 (-8.6426, 2.5111) -> (-8.7072, 2.2771) centre (0, 0) ccw
  line L320 (-8.4815, 2.3926) -> (-8.6426, 2.5111)
  arc A319 (-8.4815, 2.3926) -> (-8.5081, 2.2962) centre (0, 0) ccw
  line L321 (-8.8006, 1.8842) -> (-8.6025, 1.9122)
  arc A320 (-8.7465, 2.1209) -> (-8.8006, 1.8842) centre (0, 0) ccw
  line L322 (-8.5803, 2.0097) -> (-8.7465, 2.1209)
  arc A321 (-8.5803, 2.0097) -> (-8.6025, 1.9122) centre (0, 0) ccw
  line L323 (-8.8762, 1.4874) -> (-8.6797, 1.5243)
  arc A322 (-8.8329, 1.7263) -> (-8.8762, 1.4874) centre (0, 0) ccw
  line L324 (-8.6618, 1.6227) -> (-8.8329, 1.7263)
  arc A323 (-8.6618, 1.6227) -> (-8.6797, 1.5243) centre (0, 0) ccw
  line L325 (-8.934, 1.0877) -> (-8.7393, 1.1334)
  arc A324 (-8.9014, 1.3283) -> (-8.934, 1.0877) centre (0, 0) ccw
  line L326 (-8.7259, 1.2325) -> (-8.9014, 1.3283)
  arc A325 (-8.7259, 1.2325) -> (-8.7393, 1.1334) centre (0, 0) ccw
  line L327 (-8.9738, 0.6858) -> (-8.7814, 0.7401)
  arc A326 (-8.9521, 0.9276) -> (-8.9738, 0.6858) centre (0, 0) ccw
  line L328 (-8.7724, 0.8397) -> (-8.9521, 0.9276)
  arc A327 (-8.7724, 0.8397) -> (-8.7814, 0.7401) centre (0, 0) ccw
  arc A328 (-8.9847, 0.525) -> (-8.9956, 0.2825) centre (0, 0) ccw
  line L329 (-8.8012, 0.4453) -> (-8.9847, 0.525)
  arc A329 (-8.8012, 0.4453) -> (-8.8057, 0.3454) centre (0, 0) ccw
  line L330 (-7.3518, 5.1914) -> (-7.1587, 5.1393)
  arc A330 (-7.2091, 5.3878) -> (-7.3518, 5.1914) centre (0, 0) ccw
  line L331 (-7.5774, 4.8563) -> (-7.3821, 4.813)
  arc A331 (-7.4436, 5.0589) -> (-7.5774, 4.8563) centre (0, 0) ccw
  line L332 (-7.327, 4.8964) -> (-7.4436, 5.0589)
  arc A332 (-7.327, 4.8964) -> (-7.3821, 4.813) centre (0, 0) ccw
  line L333 (-7.7876, 4.5115) -> (-7.5906, 4.4769)
  arc A333 (-7.6631, 4.7199) -> (-7.7876, 4.5115) centre (0, 0) ccw
  line L334 (-7.5393, 4.5628) -> (-7.6631, 4.7199)
  arc A334 (-7.5393, 4.5628) -> (-7.5906, 4.4769) centre (0, 0) ccw
  line L335 (-7.9822, 4.1575) -> (-7.7838, 4.1319)
  arc A335 (-7.8671, 4.3713) -> (-7.9822, 4.1575) centre (0, 0) ccw
  line L336 (-7.7364, 4.2199) -> (-7.8671, 4.3713)
  arc A336 (-7.7364, 4.2199) -> (-7.7838, 4.1319) centre (0, 0) ccw
  line L337 (-8.1607, 3.7952) -> (-7.9614, 3.7785)
  arc A337 (-8.0553, 4.014) -> (-8.1607, 3.7952) centre (0, 0) ccw
  line L338 (-7.918, 3.8686) -> (-8.0553, 4.014)
  arc A338 (-7.918, 3.8686) -> (-7.9614, 3.7785) centre (0, 0) ccw
  line L339 (-8.3227, 3.4253) -> (-8.1229, 3.4175)
  arc A339 (-8.2273, 3.6485) -> (-8.3227, 3.4253) centre (0, 0) ccw
  line L340 (-8.0836, 3.5095) -> (-8.2273, 3.6485)
  arc A340 (-8.0836, 3.5095) -> (-8.1229, 3.4175) centre (0, 0) ccw
  line L341 (-8.468, 3.0484) -> (-8.268, 3.0496)
  arc A341 (-8.3827, 3.2757) -> (-8.468, 3.0484) centre (0, 0) ccw
  line L342 (-8.2329, 3.1433) -> (-8.3827, 3.2757)
  arc A342 (-8.2329, 3.1433) -> (-8.268, 3.0496) centre (0, 0) ccw
  line L343 (-8.5962, 2.6654) -> (-8.3965, 2.6756)
  arc A343 (-8.5212, 2.8964) -> (-8.5962, 2.6654) centre (0, 0) ccw
  line L344 (-8.3656, 2.7707) -> (-8.5212, 2.8964)
  arc A344 (-8.3656, 2.7707) -> (-8.3965, 2.6756) centre (0, 0) ccw
  line L345 (-8.7072, 2.2771) -> (-8.5081, 2.2962)
  arc A345 (-8.6426, 2.5111) -> (-8.7072, 2.2771) centre (0, 0) ccw
  line L346 (-8.4815, 2.3926) -> (-8.6426, 2.5111)
  arc A346 (-8.4815, 2.3926) -> (-8.5081, 2.2962) centre (0, 0) ccw
  line L347 (-8.8006, 1.8842) -> (-8.6025, 1.9122)
  arc A347 (-8.7465, 2.1209) -> (-8.8006, 1.8842) centre (0, 0) ccw
  line L348 (-8.5803, 2.0097) -> (-8.7465, 2.1209)
  arc A348 (-8.5803, 2.0097) -> (-8.6025, 1.9122) centre (0, 0) ccw
  line L349 (-8.8762, 1.4874) -> (-8.6797, 1.5243)
  arc A349 (-8.8329, 1.7263) -> (-8.8762, 1.4874) centre (0, 0) ccw
  line L350 (-8.6618, 1.6227) -> (-8.8329, 1.7263)
  arc A350 (-8.6618, 1.6227) -> (-8.6797, 1.5243) centre (0, 0) ccw
  line L351 (-8.934, 1.0877) -> (-8.7393, 1.1334)
  arc A351 (-8.9014, 1.3283) -> (-8.934, 1.0877) centre (0, 0) ccw
  line L352 (-8.7259, 1.2325) -> (-8.9014, 1.3283)
  arc A352 (-8.7259, 1.2325) -> (-8.7393, 1.1334) centre (0, 0) ccw
  line L353 (-8.9738, 0.6858) -> (-8.7814, 0.7401)
  arc A353 (-8.9521, 0.9276) -> (-8.9738, 0.6858) centre (0, 0) ccw
  line L354 (-8.7724, 0.8397) -> (-8.9521, 0.9276)
  arc A354 (-8.7724, 0.8397) -> (-8.7814, 0.7401) centre (0, 0) ccw
  line L355 (-8.9956, 0.2825) -> (-8.8057, 0.3454)
  arc A355 (-8.9847, 0.525) -> (-8.9956, 0.2825) centre (0, 0) ccw
  line L356 (-8.8012, 0.4453) -> (-8.9847, 0.525)
  arc A356 (-8.8012, 0.4453) -> (-8.8057, 0.3454) centre (0, 0) ccw
  line L357 (-8.9992, -0.1214) -> (-8.8124, -0.05)
  arc A357 (-8.9992, 0.1214) -> (-8.9992, -0.1214) centre (0, 0) ccw
  line L358 (-8.8124, 0.05) -> (-8.9992, 0.1214)
  arc A358 (-8.8124, 0.05) -> (-8.8124, -0.05) centre (0, 0) ccw
  line L359 (-8.9847, -0.525) -> (-8.8012, -0.4453)
  arc A359 (-8.9956, -0.2825) -> (-8.9847, -0.525) centre (0, 0) ccw
  line L360 (-8.8057, -0.3454) -> (-8.9956, -0.2825)
  arc A360 (-8.8057, -0.3454) -> (-8.8012, -0.4453) centre (0, 0) ccw
  line L361 (-8.9521, -0.9276) -> (-8.7724, -0.8397)
  arc A361 (-8.9738, -0.6858) -> (-8.9521, -0.9276) centre (0, 0) ccw
  line L362 (-8.7814, -0.7401) -> (-8.9738, -0.6858)
  arc A362 (-8.7814, -0.7401) -> (-8.7724, -0.8397) centre (0, 0) ccw
  line L363 (-8.9014, -1.3283) -> (-8.7259, -1.2325)
  arc A363 (-8.934, -1.0877) -> (-8.9014, -1.3283) centre (0, 0) ccw
  line L364 (-8.7393, -1.1334) -> (-8.934, -1.0877)
  arc A364 (-8.7393, -1.1334) -> (-8.7259, -1.2325) centre (0, 0) ccw
  line L365 (-8.8329, -1.7263) -> (-8.6618, -1.6227)
  arc A365 (-8.8762, -1.4874) -> (-8.8329, -1.7263) centre (0, 0) ccw
  line L366 (-8.6797, -1.5243) -> (-8.8762, -1.4874)
  arc A366 (-8.6797, -1.5243) -> (-8.6618, -1.6227) centre (0, 0) ccw
  line L367 (-8.7465, -2.1209) -> (-8.5803, -2.0097)
  arc A367 (-8.8006, -1.8842) -> (-8.7465, -2.1209) centre (0, 0) ccw
  line L368 (-8.6025, -1.9122) -> (-8.8006, -1.8842)
  arc A368 (-8.6025, -1.9122) -> (-8.5803, -2.0097) centre (0, 0) ccw
  line L369 (-8.6426, -2.5111) -> (-8.4815, -2.3926)
  arc A369 (-8.7072, -2.2771) -> (-8.6426, -2.5111) centre (0, 0) ccw
  line L370 (-8.5081, -2.2962) -> (-8.7072, -2.2771)
  arc A370 (-8.5081, -2.2962) -> (-8.4815, -2.3926) centre (0, 0) ccw
  line L371 (-8.5212, -2.8964) -> (-8.3656, -2.7707)
  arc A371 (-8.5962, -2.6654) -> (-8.5212, -2.8964) centre (0, 0) ccw
  line L372 (-8.3965, -2.6756) -> (-8.5962, -2.6654)
  arc A372 (-8.3965, -2.6756) -> (-8.3656, -2.7707) centre (0, 0) ccw
  line L373 (-8.3827, -3.2757) -> (-8.2329, -3.1433)
  arc A373 (-8.468, -3.0484) -> (-8.3827, -3.2757) centre (0, 0) ccw
  line L374 (-8.268, -3.0496) -> (-8.468, -3.0484)
  arc A374 (-8.268, -3.0496) -> (-8.2329, -3.1433) centre (0, 0) ccw
  line L375 (-8.2273, -3.6485) -> (-8.0836, -3.5095)
  arc A375 (-8.3227, -3.4253) -> (-8.2273, -3.6485) centre (0, 0) ccw
  line L376 (-8.1229, -3.4175) -> (-8.3227, -3.4253)
  arc A376 (-8.1229, -3.4175) -> (-8.0836, -3.5095) centre (0, 0) ccw
  line L377 (-8.0553, -4.014) -> (-7.918, -3.8686)
  arc A377 (-8.1607, -3.7952) -> (-8.0553, -4.014) centre (0, 0) ccw
  line L378 (-7.9614, -3.7785) -> (-8.1607, -3.7952)
  arc A378 (-7.9614, -3.7785) -> (-7.918, -3.8686) centre (0, 0) ccw
  line L379 (-7.8671, -4.3713) -> (-7.7364, -4.2199)
  arc A379 (-7.9822, -4.1575) -> (-7.8671, -4.3713) centre (0, 0) ccw
  line L380 (-7.7838, -4.1319) -> (-7.9822, -4.1575)
  arc A380 (-7.7838, -4.1319) -> (-7.7364, -4.2199) centre (0, 0) ccw
  line L381 (-7.6631, -4.7199) -> (-7.5393, -4.5628)
  arc A381 (-7.7876, -4.5115) -> (-7.6631, -4.7199) centre (0, 0) ccw
  line L382 (-7.5906, -4.4769) -> (-7.7876, -4.5115)
  arc A382 (-7.5906, -4.4769) -> (-7.5393, -4.5628) centre (0, 0) ccw
  line L383 (-7.4436, -5.0589) -> (-7.327, -4.8964)
  arc A383 (-7.5774, -4.8563) -> (-7.4436, -5.0589) centre (0, 0) ccw
  line L384 (-7.3821, -4.813) -> (-7.5774, -4.8563)
  arc A384 (-7.3821, -4.813) -> (-7.327, -4.8964) centre (0, 0) ccw
  arc A385 (-7.3518, -5.1914) -> (-7.2091, -5.3878) centre (0, 0) ccw
  line L385 (-7.1587, -5.1393) -> (-7.3518, -5.1914)
  circle A386 centre (0, 0) radius 6.25
  circle A387 centre (0, 0) radius 9
  point P0 (6.6364, 5.7981)
  point P1 (6.3696, 6.09)
  point P2 (6.09, 6.3696)
  point P3 (5.7981, 6.6364)
  point P4 (5.4945, 6.8899)
  point P5 (5.1799, 7.1295)
  point P6 (4.8548, 7.3547)
  point P7 (4.5199, 7.5651)
  point P8 (4.176, 7.7602)
  point P9 (3.8236, 7.9398)
  point P10 (3.4635, 8.1033)
  point P11 (3.0965, 8.2506)
  point P12 (2.7232, 8.3812)
  point P13 (2.3444, 8.4949)
  point P14 (1.961, 8.5916)
  point P15 (1.5735, 8.6709)
  point P16 (1.1829, 8.7327)
  point P17 (0.7899, 8.777)
  point P18 (0.3954, 8.8036)
  point P19 (0, 8.8125)
  point P20 (-0.3954, 8.8036)
  point P21 (-0.7899, 8.777)
  point P22 (-1.1829, 8.7327)
  point P23 (-1.5735, 8.6709)
  point P24 (-1.961, 8.5916)
  point P25 (-2.3444, 8.4949)
  point P26 (-2.7232, 8.3812)
  point P27 (-3.0965, 8.2506)
  point P28 (-3.4635, 8.1033)
  point P29 (-3.8236, 7.9398)
  point P30 (-4.176, 7.7602)
  point P31 (-4.5199, 7.5651)
  point P32 (-4.8548, 7.3547)
  point P33 (-5.1799, 7.1295)
  point P34 (-5.4945, 6.8899)
  point P35 (-5.7981, 6.6364)
  point P36 (-6.09, 6.3696)
  point P37 (-6.3696, 6.09)
  point P38 (-6.6364, 5.7981)
  point P39 (7.3547, -4.8548)
  point P40 (7.5651, -4.5199)
  point P41 (7.7602, -4.176)
  point P42 (7.9398, -3.8236)
  point P43 (8.1033, -3.4635)
  point P44 (8.2506, -3.0965)
  point P45 (8.3812, -2.7232)
  point P46 (8.4949, -2.3444)
  point P47 (8.5916, -1.961)
  point P48 (8.6709, -1.5735)
  point P49 (8.7327, -1.1829)
  point P50 (8.777, -0.7899)
  point P51 (8.8036, -0.3954)
  point P52 (8.8125, 0)
  point P53 (8.8036, 0.3954)
  point P54 (8.777, 0.7899)
  point P55 (8.7327, 1.1829)
  point P56 (8.6709, 1.5735)
  point P57 (8.5916, 1.961)
  point P58 (8.4949, 2.3444)
  point P59 (8.3812, 2.7232)
  point P60 (8.2506, 3.0965)
  point P61 (8.1033, 3.4635)
  point P62 (7.9398, 3.8236)
  point P63 (7.7602, 4.176)
  point P64 (7.5651, 4.5199)
  point P65 (7.3547, 4.8548)
  point P66 (7.1295, 5.1799)
  point P67 (6.8899, 5.4945)
  point P68 (6.6364, 5.7981)
  point P69 (6.3696, 6.09)
  point P70 (6.09, 6.3696)
  point P71 (5.7981, 6.6364)
  point P72 (5.4945, 6.8899)
  point P73 (5.1799, 7.1295)
  point P74 (4.8548, 7.3547)
  point P75 (4.5199, 7.5651)
  point P76 (4.176, 7.7602)
  point P77 (3.8236, 7.9398)
  point P78 (1.5735, -8.6709)
  point P79 (1.961, -8.5916)
  point P80 (2.3444, -8.4949)
  point P81 (2.7232, -8.3812)
  point P82 (3.0965, -8.2506)
  point P83 (3.4635, -8.1033)
  point P84 (3.8236, -7.9398)
  point P85 (4.176, -7.7602)
  point P86 (4.5199, -7.5651)
  point P87 (4.8548, -7.3547)
  point P88 (5.1799, -7.1295)
  point P89 (5.4945, -6.8899)
  point P90 (5.7981, -6.6364)
  point P91 (6.09, -6.3696)
  point P92 (6.3696, -6.09)
  point P93 (6.6364, -5.7981)
  point P94 (6.8899, -5.4945)
  point P95 (7.1295, -5.1799)
  point P96 (7.3547, -4.8548)
  point P97 (7.5651, -4.5199)
  point P98 (7.7602, -4.176)
  point P99 (7.9398, -3.8236)
  point P100 (8.1033, -3.4635)
  point P101 (8.2506, -3.0965)
  point P102 (8.3812, -2.7232)
  point P103 (8.4949, -2.3444)
  point P104 (8.5916, -1.961)
  point P105 (8.6709, -1.5735)
  point P106 (8.7327, -1.1829)
  point P107 (8.777, -0.7899)
  point P108 (8.8036, -0.3954)
  point P109 (8.8125, 0)
  point P110 (0.3954, -8.8036)
  point P111 (0.7899, -8.777)
  point P112 (1.1829, -8.7327)
  point P113 (1.5735, -8.6709)
  point P114 (1.961, -8.5916)
  point P115 (2.3444, -8.4949)
  point P116 (-8.1033, -3.4635)
  point P117 (-7.9398, -3.8236)
  point P118 (-7.7602, -4.176)
  point P119 (-7.5651, -4.5199)
  point P120 (-7.3547, -4.8548)
  point P121 (-7.1295, -5.1799)
  point P122 (-6.8899, -5.4945)
  point P123 (-6.6364, -5.7981)
  point P124 (-6.3696, -6.09)
  point P125 (-6.09, -6.3696)
  point P126 (-5.7981, -6.6364)
  point P127 (-5.4945, -6.8899)
  point P128 (-5.1799, -7.1295)
  point P129 (-4.8548, -7.3547)
  point P130 (-4.5199, -7.5651)
  point P131 (-4.176, -7.7602)
  point P132 (-3.8236, -7.9398)
  point P133 (-3.4635, -8.1033)
  point P134 (-3.0965, -8.2506)